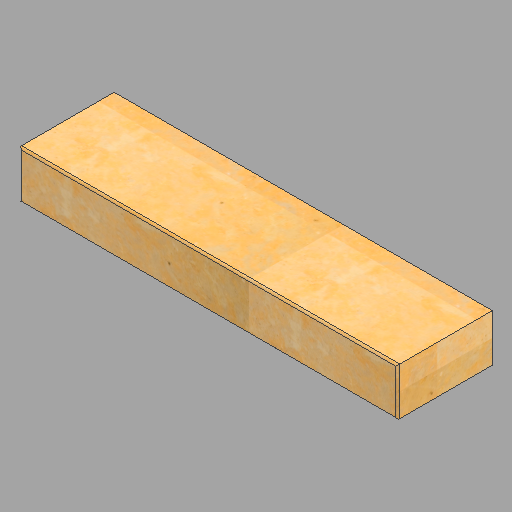
# Autodesk Inventor part: 6in-511LF
Saved by Autodesk Inventor 2023 (Build 270158030, 158C)
## iProperties
RuleStatus: InUse
Created: 2022-09-15
Part Number: 6in-511LF
Material: Granite, Cut, Polished
Document SubType Name: Modeling
Designer: awelt
Mass: 152868 g
Surface Area: 12019 cm^2
Volume: 56617.9 cm^3
Density: 2.7 g/cm^3
Appearance: Amber Select
AfterDocSave0: Convert in3 volume to ft3
in3 to ft3: 0.0
TEST: 0.001
Author: awelt
Autodesk Inventor part; units mm, degrees
ref_plane "YZ Plane" through (0, 0, 0) normal (1, 0, 0) x (0, 1, 0)
ref_plane "XZ Plane" through (0, 0, 0) normal (0, 1, 0) x (-1, 0, 0)
ref_plane "XY Plane" through (0, 0, 0) normal (0, 0, 1) x (1, 0, 0)
sketch "Sketch1" plane through (0, 0, 0) normal (1, 0, 0) x (0, 1, 0)
  line L0 (0, 0) -> (152.4, 0)
  line L1 (152.4, 0) -> (152.4, 254)
  line L2 (152.4, 254) -> (0, 254)
  line L3 (0, 254) -> (0, 0)
  dimension "d0" = 152.4
  dimension "d1" = 254
  constraints: 8 end point, 2 parallel, 1 horizontal, 1 perpendicular
  measures "d0" distance of L2.end L1.end
  measures "d1" distance of L1.end L0.end
extrude "Extrusion1" add sketch "Sketch1" along normal blind 1219.2
fillet "Fillet1" radius 6.35 3 edges at (609.6, 152.4, 254) (1219.2, 76.2, 254) (0, 76.2, 254)
fillet "Fillet2" radius 3.175 1 edges at (609.6, 0, 254)
move faces "Move1" translate (0, 0, -50.8) faces at (406.4, 50.8, 0)
body "Solid1"
